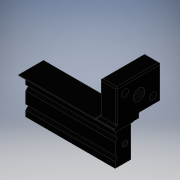
# Autodesk Inventor part: SCHUNK-5521119 Finger EGP 40
Saved by Autodesk Inventor 2019 (Build 230136000, 136)
## iProperties
Created: 2022-08-29
Part Number: SCHUNK-5521119 Finger EGP 40
Material: Generic
Catalog Web Link: www.cadenas.de
Description: EGP-Electrical 2-finger parallel gripper
Vendor: SCHUNK
Document SubType Name: Modeling
Designer: psAdmin
Manufacturer: SCHUNK
Mass: 3.36917 g
Surface Area: 24.5799 cm^2
Volume: 3.36917 cm^3
Density: 1 g/cm^3
Appearance: PSOLRGB-51-51-51
Category: PARTsolutions
Company: SCHUNK
Title: SCHUNK-5521119 Finger EGP 40
Author: Cadenas PARTsolutions
Comments: Electrical 2-finger parallel gripper
PSOL_IDENT_0: {$CADENAS_DATA/23d-libs/schunk/greifsysteme/greifmodule/greifmodule_elektrisch/2_finger_parallelgrei
PSOL_IDENT_1: fer/kleinteilegreifer/egp/egp_fin.prj},193 {VTYP=3D},{NB=SCHUNK-5521119 Finger EGP 40},{LINA=SCHUNK-
PSOL_IDENT_2: 5521119 Finger EGP 40},{NN=EGP},{DATE=27.06.2022 11:10:53},{GEOMDATE=15.04.2020 08:38:29},{VERSION=}
PSOL_IDENT_3: ,{LINEID=20},{WBVAR=},{WBNUMERIC=}  {NB=SCHUNK-5521119 Finger EGP 40},{LINA=SCHUNK-5521119 Finger EG
PSOL_IDENT_4: P 40},{KT=DUMMY},{IDNR=5521119},{TYP=EGP 40},{TYP1=2.000},{LGES=34.000},{BGES=17.000},{HGES=25.600},
PSOL_IDENT_5: {B1=9.950},{H1=12.400},{B2=8.100},{H2=14.100},{F1=0.300},{B3=15.500},{H3=12.200},{B4=16.000},{H4=13.
PSOL_IDENT_6: 300},{L1=3.000},{L2=6.000},{T1=0.900},{H5=12.200},{L3=1.000},{L4=6.000},{R1=0.800},{F2=0.800},{F10=0
PSOL_IDENT_7: .500},{D1=5.000},{L5=6.000},{D2=2.500},{L6=10.000},{L7=6.000},{D3=2.500},{T3=5.500},{T4=7.500},{L8=6
PSOL_IDENT_8: .000},{L9=12.000},{CNSCTN=84798997}
NB: SCHUNK-5521119 Finger EGP 40
NN: EGP
NT: Electrical 2-finger parallel gripper
NBSYN: SCHUNK-$IDNR. Finger $TYP.
LINA: SCHUNK-5521119 Finger EGP 40
CATALOG: SCHUNK
IDNR: 5521119
TYP: EGP 40
TYP1: 2
LGES: 34
BGES: 17
HGES: 25.6
B1: 9.95
H1: 12.4
B2: 8.1
H2: 14.1
F1: 0.3
B3: 15.5
H3: 12.2
B4: 16
H4: 13.3
L1: 3
L2: 6
T1: 0.9
H5: 12.2
L3: 1
L4: 6
R1: 0.8
F2: 0.8
F10: 0.5
D1: 5
L5: 6
D2: 2.5
L6: 10
L7: 6
D3: 2.5
T3: 5.5
T4: 7.5
L8: 6
L9: 12
CNSCTN: 84798997
SUPPLIER: SCHUNK
ARTICLENO: SCHUNK-5521119 Finger EGP 40
BOMINFO: SCHUNK-5521119 Finger EGP 40
CREATOR: CADENAS GmbH
Autodesk Inventor part; units mm, degrees
sketch "Sketch_1" plane through (0, 0, 0) normal (1, 0, 0) x (0, 1, 0)
  line L0 (-12.3, 9) -> (-12.6, 9)
  line L1 (-12.6, 9) -> (-13.4, 8.2)
  line L2 (-13.4, 8.2) -> (-13.4, 7.5)
  line L3 (-13.4, 7.5) -> (-25.6, 7.5)
  line L4 (-25.6, 7.5) -> (-25.6, 1.95)
  line L5 (-25.6, 1.95) -> (-13.2, 1.95)
  line L6 (-13.2, 1.95) -> (-13.2, 0.1)
  line L7 (-13.2, 0.1) -> (-11.8, 0.1)
  line L8 (-11.8, 0.1) -> (-11.5, -0.2)
  line L9 (-11.5, -0.2) -> (-11.5, -8)
  line L10 (-11.5, -8) -> (-0.5, -8)
  line L11 (-0.5, -8) -> (0, -7.5)
  line L12 (0, -7.5) -> (0, 7.5)
  line L13 (0, 7.5) -> (-0.5, 8)
  line L14 (-0.5, 8) -> (-11.5, 8)
  arc A0 (-12.3, 8.8) -> (-11.5, 8) centre (-11.5, 8.8) ccw
  line L15 (-12.3, 8.8) -> (-12.3, 9)
  constraints: 32 end point, 2 point on circle, 1 centre point
extrude "Extrusion1" add sketch "Sketch_1" against normal blind 34
sketch "Sketch_2" plane through (0, 0, 0) normal (0, 0, 1) x (1, 0, 0)
  line L0 (-35, 1) -> (-35, -26.6)
  line L1 (-35, -26.6) -> (0, -26.6)
  line L2 (0, -26.6) -> (0, -13.4)
  line L3 (0, -13.4) -> (-1, -13.4)
  line L4 (-1, -13.4) -> (-1, -25.6)
  line L5 (-1, -25.6) -> (-33, -25.6)
  line L6 (-33, -25.6) -> (-33, -13.4)
  line L7 (-33, -13.4) -> (-34, -13.4)
  line L8 (-34, -13.4) -> (-34, -12.3)
  line L9 (-34, -12.3) -> (-6.8, -12.3)
  arc A0 (-6.8, -12.3) -> (-6, -11.5) centre (-6.8, -11.5) ccw
  line L10 (-6, -11.5) -> (-6, -0.5)
  line L11 (-6, -0.5) -> (-5.5, 0)
  line L12 (-5.5, 0) -> (-0.5, 0)
  line L13 (-0.5, 0) -> (0, -0.5)
  line L14 (0, -0.5) -> (0, 1)
  line L15 (0, 1) -> (-35, 1)
  constraints: 32 end point, 2 point on circle, 1 centre point
extrude "Extrusion2" cut sketch "Sketch_2" along normal mid plane 68
sketch "Sketch_3" plane through (0, 0, 0) normal (0, 1, 0) x (-1, 0, 0)
  circle A0 centre (0, 0) radius 34
  line L0 (6, -7.5) -> (6, 7.5)
  line L1 (6, 7.5) -> (5.5, 8)
  line L2 (5.5, 8) -> (0.5, 8)
  line L3 (0.5, 8) -> (0, 7.5)
  line L4 (0, 7.5) -> (0, -7.5)
  line L5 (0, -7.5) -> (0.5, -8)
  line L6 (0.5, -8) -> (5.5, -8)
  line L7 (5.5, -8) -> (6, -7.5)
  constraints: 16 end point, 1 centre point
extrude "Extrusion3" cut sketch "Sketch_3" against normal blind 11.5
sketch "Sketch_4" plane through (0, 0, 0) normal (1, 0, 0) x (0, 1, 0)
  line L0 (-14.7, 8.5) -> (-24.5, 8.5)
  line L1 (-24.5, 8.5) -> (-22.6, 6.6)
  line L2 (-22.6, 6.6) -> (-21.7, 7.5)
  line L3 (-21.7, 7.5) -> (-17.5, 7.5)
  line L4 (-17.5, 7.5) -> (-16.6, 6.6)
  line L5 (-16.6, 6.6) -> (-14.7, 8.5)
  constraints: 12 end point
extrude "Extrusion4" cut sketch "Sketch_4" against normal blind 34
sketch "Sketch5" plane through (-6, -11.5, 7.5) normal (-1, 0, 0) x (0, 0, 1)
  point P0 (-7.5, 5.5)
hole "Hole1" at (-6, -6, 0) direction (1, 0, 0) diameter 4.134 depth 6 thread size "M5x0.8" class "6H" standard "ISO Metric profile"
sketch "Sketch6" plane through (0, 0, 0) normal (1, 0, 0) x (0, 0, -1)
  point P0 (-5, -3)
hole "Hole2" at (0, -3, 5) direction (-1, 0, 0) diameter 2.5 depth 6
pattern_linear "Rectangular Pattern1" count 2 spacing 11.6619 along (0, -0.5145, -0.8575) of "Hole2"
sketch "Sketch7" plane through (-1, -25.6, 1.95) normal (1, 0, 0) x (0, 0, -1)
  point P0 (-2.05, 6)
hole "Hole3" at (-1, -19.6, 4) direction (-1, 0, 0) diameter 2.013 depth 7.5 tip angle 121 thread size "M2.5x0.45" class "6H" standard "ISO Metric profile"
sketch "Sketch8" plane through (-33, -25.6, 1.95) normal (-1, 0, 0) x (0, 0, 1)
  point P0 (2.05, 6)
hole "Hole4" at (-33, -19.6, 4) direction (1, 0, 0) diameter 2.013 depth 7.5 tip angle 121 thread size "M2.5x0.45" class "6H" standard "ISO Metric profile"
ref_plane "HUB_XY" through (-6, 0, 0) normal (1, 0, 0) x (0, 0, -1)
ref_plane "HUB_YZ" through (-6, 0, 0) normal (0, 0, -1) x (0, 1, 0)
ref_plane "HUB_ZX" through (-6, 0, 0) normal (0, 1, 0) x (1, 0, 0)
ref_plane "hal_1_XY" through (-1, -19.6, 4) normal (1, 0, 0) x (0, 0, -1)
ref_plane "hal_1_YZ" through (-1, -19.6, 4) normal (0, 0, -1) x (0, 1, 0)
ref_plane "hal_1_ZX" through (-1, -19.6, 4) normal (0, 1, 0) x (1, 0, 0)
ref_plane "hal_2_XY" through (-33, -19.6, 4) normal (1, 0, 0) x (0, 0, -1)
ref_plane "hal_2_YZ" through (-33, -19.6, 4) normal (0, 0, -1) x (0, 1, 0)
ref_plane "hal_2_ZX" through (-33, -19.6, 4) normal (0, 1, 0) x (1, 0, 0)
body "Solid1"
